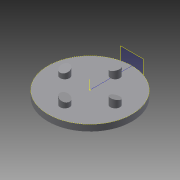
# Autodesk Inventor part: innerbaycon4
Saved by Autodesk Inventor 2015 (Build 190159000, 159)
## iProperties
Created: 2014-12-03
Part Number: innerbaycon4
Material: Generic
Document SubType Name: Modeling
Designer: ericd_000
Density: 1 g/cm^3
Appearance: Default
Author: ericd_000
Autodesk Inventor part; units mm, degrees
ref_plane "YZ Plane" through (0, 0, 0) normal (1, 0, 0) x (0, 1, 0)
ref_plane "XZ Plane" through (0, 0, 0) normal (0, 1, 0) x (-1, 0, 0)
ref_plane "XY Plane" through (0, 0, 0) normal (0, 0, 1) x (1, 0, 0)
sketch "Sketch1" plane through (0, 0, 0) normal (0, 0, 1) x (1, 0, 0)
  circle A0 centre (0, 0) radius 40
  dimension "d0" = 80
  constraints: 1 centre point, 1 coincident
  measures "d0" diameter of A0
extrude "Extrusion1" add sketch "Sketch1" along normal blind 6
sketch "Sketch2" plane through (0, 0, 6) normal (0, 0, 1) x (1, 0, 0)
  circle A0 centre (0, 24) radius 4.5
  point P0 (0, 0)
  dimension "d3" = 9
  dimension "d4" = 24
  constraints: 1 centre point
  measures "d3" diameter of A0
  measures "d4" distance of point (0, 0) A0.centre
extrude "Extrusion2" add sketch "Sketch2" along normal blind 7.5
sketch "Sketch3" plane through (0, 0, 6) normal (0, 0, 1) x (1, 0, 0)
  line L0 (0, 0) -> (0, 40) construction
  circle A0 centre (0, 0) radius 40 construction
  constraints: 2 end point, 1 vertical, 1 vertical alignment, 1 other
ref_plane "Work Plane1" through (0, 40, 6) normal (0, 1, 0) x (-1, 0, 0)
sketch "Sketch4" plane through (0, 40, 6) normal (0, 1, 0) x (-1, 0, 0)
  line L0 (-4.5029, 7.5) -> (4.4959, 7.5)
  line L1 (4.5, 7.5) -> (-4.5, 7.5) projected
  line L2 (-4.5, 0) -> (-4.5, 7.5) projected
  line L3 (4.5, 7.5) -> (4.5, 4.5)
  line L4 (4.5, 4.5) -> (-4.5, 7.5)
  point P0 (0, -6)
  dimension "d12" = 3
  constraints: 6 end point, 1 point on line, 1 vertical
  measures "d12" distance of L1.start L3.end
extrude "Extrusion3" cut sketch "Sketch4" against normal blind 25
pattern_circular "Circular Pattern1" count 4 over 360 about axis through (0, 0, 0) along (0, 0, 1) of "Extrusion2", "Extrusion3"
body "Solid1"
